Autodesk Inventor part; units mm, degrees
(part 2 of 2)
sketch "スケッチ3" plane through (0, 0, 0) normal (0, 0, 1) x (1, 0, 0)
  circle A0 centre (-65.3767, 79.8352) radius 5.25 projected
  arc A1 (-43.2653, 88.6866) -> (-43.9344, 87.9435) centre (-42.9563, 87.7355) ccw projected
  line L0 (-43.9344, 87.9435) -> (-47.1214, 72.9516) projected
  arc A2 (-47.1214, 72.9516) -> (-45.8786, 71.7794) centre (-46.1433, 72.7437) ccw projected
  arc A3 (-42.2436, 64.1319) -> (-45.8786, 71.7794) centre (-44.7404, 67.6327) ccw projected
  arc A4 (-42.2436, 64.1319) -> (-42.659, 63.2293) centre (-41.663, 63.3177) ccw projected
  arc A5 (-53.0468, 54.5405) -> (-42.659, 63.2293) centre (-50.8767, 62.5) ccw projected
  arc A6 (-53.0468, 54.5405) -> (-54.0085, 54.2911) centre (-53.3098, 53.5757) ccw projected
  arc A7 (-59.6272, 53.9531) -> (-54.0085, 54.2911) centre (-57.0131, 57.3673) ccw projected
  arc A8 (-59.6272, 53.9531) -> (-60.795, 53.9877) centre (-60.2351, 53.1591) ccw projected
  line L1 (-60.795, 53.9877) -> (-61.9497, 53.2074) projected
  arc A9 (-61.9497, 53.2074) -> (-62.3865, 52.4596) centre (-61.3898, 52.3788) ccw projected
  arc A10 (-68.3669, 52.4596) -> (-62.3865, 52.4596) centre (-65.3767, 52.702) ccw projected
  arc A11 (-68.3669, 52.4596) -> (-68.8038, 53.2074) centre (-69.3637, 52.3788) ccw projected
  line L2 (-68.8038, 53.2074) -> (-69.9585, 53.9877) projected
  arc A12 (-69.9585, 53.9877) -> (-71.1263, 53.9531) centre (-70.5184, 53.1591) ccw projected
  arc A13 (-76.7449, 54.2911) -> (-71.1263, 53.9531) centre (-73.7404, 57.3673) ccw projected
  arc A14 (-76.7449, 54.2911) -> (-77.7067, 54.5405) centre (-77.4437, 53.5757) ccw projected
  arc A15 (-88.0944, 63.2293) -> (-77.7067, 54.5405) centre (-79.8767, 62.5) ccw projected
  arc A16 (-88.0944, 63.2293) -> (-88.5099, 64.1319) centre (-89.0905, 63.3177) ccw projected
  arc A17 (-89.8355, 69.6024) -> (-88.5099, 64.1319) centre (-86.0131, 67.6327) ccw projected
  arc A18 (-89.8355, 69.6024) -> (-90.0078, 70.7579) centre (-90.7244, 70.0604) ccw projected
  line L3 (-90.0078, 70.7579) -> (-90.9798, 71.7565) projected
  arc A19 (-90.9798, 71.7565) -> (-91.7931, 72.0544) centre (-91.6964, 71.059) ccw projected
  arc A20 (-92.8499, 77.9406) -> (-91.7931, 72.0544) centre (-92.0829, 75.0403) ccw projected
  arc A21 (-92.8499, 77.9406) -> (-92.1911, 78.5027) centre (-93.1056, 78.9074) ccw projected
  line L4 (-92.1911, 78.5027) -> (-91.6272, 79.7771) projected
  arc A22 (-91.6272, 79.7771) -> (-91.8676, 80.9205) centre (-92.5416, 80.1818) ccw projected
  arc A23 (-92.5278, 86.5104) -> (-91.8676, 80.9205) centre (-88.9691, 84.0968) ccw projected
  arc A24 (-92.5278, 86.5104) -> (-92.4523, 87.5011) centre (-93.3554, 87.0717) ccw projected
  arc A25 (-85.7359, 99.2608) -> (-92.4523, 87.5011) centre (-85.0015, 91.0436) ccw projected
  arc A26 (-85.7359, 99.2608) -> (-84.921, 99.8292) centre (-85.8249, 100.2569) ccw projected
  arc A27 (-79.7708, 102.1007) -> (-84.921, 99.8292) centre (-81.034, 97.9904) ccw projected
  arc A28 (-79.7708, 102.1007) -> (-78.6639, 102.4745) centre (-79.4771, 103.0566) ccw projected
  line L5 (-78.6639, 102.4745) -> (-77.8528, 103.6077) projected
  arc A29 (-77.8528, 103.6077) -> (-77.7034, 104.4608) centre (-78.6659, 104.1898) ccw projected
  arc A30 (-72.0965, 106.5412) -> (-77.7034, 104.4608) centre (-74.8156, 105.2737) ccw projected
  arc A31 (-72.0965, 106.5412) -> (-71.4268, 105.9921) centre (-71.1901, 106.9637) ccw projected
  line L6 (-71.4268, 105.9921) -> (-70.0728, 105.6623) projected
  arc A32 (-70.0728, 105.6623) -> (-68.99, 106.1009) centre (-69.8361, 106.6338) ccw projected
  arc A33 (-63.6047, 107.7386) -> (-68.99, 106.1009) centre (-65.3514, 103.8094) ccw projected
  arc A34 (-63.6047, 107.7386) -> (-62.6162, 107.8393) centre (-63.1984, 108.6523) ccw projected
  arc A35 (-49.8547, 103.3068) -> (-62.6162, 107.8393) centre (-57.8128, 101.1319) ccw projected
  arc A36 (-49.8547, 103.3068) -> (-49.1512, 102.6051) centre (-48.89, 103.5704) ccw projected
  arc A37 (-46.0508, 97.6465) -> (-49.1512, 102.6051) centre (-50.2742, 98.4544) ccw projected
  arc A38 (-46.0508, 97.6465) -> (-44.9551, 96.465) centre (-45.0686, 97.4586) ccw projected
  arc A39 (-43.2653, 88.6866) -> (-44.9551, 96.465) centre (-44.5012, 92.4909) ccw projected
  arc A40 (-60.3905, 85.4377) -> (-59.2073, 85.3296) centre (-59.7257, 86.1847) ccw projected
  line L7 (-59.2073, 85.3296) -> (-48.9817, 91.5288) projected
  arc A41 (-48.9817, 91.5288) -> (-48.5003, 92.4053) centre (-49.5001, 92.3839) ccw projected
  arc A42 (-48.4958, 92.6994) -> (-48.5003, 92.4053) centre (-44.5012, 92.4909) ccw projected
  arc A43 (-48.4958, 92.6994) -> (-48.95, 93.5904) centre (-49.4944, 92.7516) ccw projected
  line L8 (-48.95, 93.5904) -> (-49.574, 93.9954) projected
  arc A44 (-49.574, 93.9954) -> (-50.1478, 94.1562) centre (-50.1185, 93.1567) ccw projected
  arc A45 (-52.021, 94.5252) -> (-50.1478, 94.1562) centre (-50.2742, 98.4544) ccw projected
  arc A46 (-52.021, 94.5252) -> (-53.0094, 94.4244) centre (-52.4272, 93.6114) ccw projected
  arc A47 (-65.771, 98.9569) -> (-53.0094, 94.4244) centre (-57.8128, 101.1319) ccw projected
  arc A48 (-65.771, 98.9569) -> (-66.4744, 99.6586) centre (-66.7356, 98.6933) ccw projected
  arc A49 (-69.2468, 101.9882) -> (-66.4744, 99.6586) centre (-65.3514, 103.8094) ccw projected
  arc A50 (-69.2468, 101.9882) -> (-69.916, 102.5363) centre (-70.1527, 101.5647) ccw projected
  line L9 (-69.916, 102.5363) -> (-70.5978, 102.7024) projected
  arc A51 (-70.5978, 102.7024) -> (-71.772, 101.383) centre (-70.8345, 101.7308) ccw projected
  line L10 (-71.772, 101.383) -> (-66.7965, 87.9737) projected
  arc A52 (-66.7965, 87.9737) -> (-65.8023, 87.3231) centre (-65.859, 88.3215) ccw projected
  arc A53 (-60.3905, 85.4377) -> (-65.8023, 87.3231) centre (-65.3767, 79.8352) ccw projected
  line L11 (-63.8767, 71.7112) -> (-63.8767, 57.4086) projected
  arc A54 (-63.8767, 57.4086) -> (-62.3169, 56.58) centre (-62.8767, 57.4086) ccw projected
  line L12 (-62.3169, 56.58) -> (-61.7354, 56.9729) projected
  arc A55 (-61.7354, 56.9729) -> (-61.2986, 57.7196) centre (-62.2953, 57.8015) ccw projected
  arc A56 (-59.5099, 60.8681) -> (-61.2986, 57.7196) centre (-57.0131, 57.3673) ccw projected
  arc A57 (-59.5099, 60.8681) -> (-59.0944, 61.7707) centre (-60.0905, 61.6823) ccw projected
  arc A58 (-51.4061, 70.733) -> (-59.0944, 61.7707) centre (-50.8767, 62.5) ccw projected
  arc A59 (-51.4061, 70.733) -> (-50.4921, 71.523) centre (-51.4703, 71.7309) ccw projected
  line L13 (-50.4921, 71.523) -> (-47.1705, 87.1482) projected
  arc A60 (-47.1705, 87.1482) -> (-48.6671, 88.2112) centre (-48.1487, 87.3561) ccw projected
  line L14 (-48.6671, 88.2112) -> (-58.3104, 82.365) projected
  arc A61 (-58.3494, 82.4556) -> (-58.3104, 82.365) centre (-57.4124, 82.805) ccw projected
  arc A62 (-63.1709, 72.667) -> (-58.3494, 82.4556) centre (-65.3767, 79.8352) ccw projected
  arc A63 (-63.1709, 72.667) -> (-63.8767, 71.7112) centre (-62.8767, 71.7112) ccw projected
  line L15 (-66.8767, 57.4086) -> (-66.8767, 71.7112) projected
  arc A64 (-66.8767, 71.7112) -> (-67.5826, 72.667) centre (-67.8767, 71.7112) ccw projected
  arc A65 (-72.0424, 76.3973) -> (-67.5826, 72.667) centre (-65.3767, 79.8352) ccw projected
  arc A66 (-72.0424, 76.3973) -> (-73.1078, 76.9232) centre (-72.9311, 75.9389) ccw projected
  line L16 (-73.1078, 76.9232) -> (-87.1853, 74.3957) projected
  arc A67 (-87.1853, 74.3957) -> (-87.7252, 72.7139) centre (-87.0086, 73.4114) ccw projected
  line L17 (-87.7252, 72.7139) -> (-87.2357, 72.211) projected
  arc A68 (-87.2357, 72.211) -> (-86.4237, 71.9131) centre (-86.5192, 72.9085) ccw projected
  arc A69 (-83.0085, 70.7089) -> (-86.4237, 71.9131) centre (-86.0131, 67.6327) ccw projected
  arc A70 (-83.0085, 70.7089) -> (-82.0468, 70.4595) centre (-82.3098, 71.4243) ccw projected
  arc A71 (-71.659, 61.7707) -> (-82.0468, 70.4595) centre (-79.8767, 62.5) ccw projected
  arc A72 (-71.659, 61.7707) -> (-71.2436, 60.8681) centre (-70.663, 61.6823) ccw projected
  arc A73 (-69.4548, 57.7196) -> (-71.2436, 60.8681) centre (-73.7404, 57.3673) ccw projected
  arc A74 (-69.4548, 57.7196) -> (-69.0181, 56.9729) centre (-68.4582, 57.8015) ccw projected
  line L18 (-69.0181, 56.9729) -> (-68.4366, 56.58) projected
  arc A75 (-68.4366, 56.58) -> (-66.8767, 57.4086) centre (-67.8767, 57.4086) ccw projected
  circle A76 centre (-74.8156, 105.2737) radius 1.5 projected
  circle A77 centre (-92.0829, 75.0403) radius 1.5 projected
  circle A78 centre (-85.0015, 91.0436) radius 5.25 projected
  circle A79 centre (-88.9691, 84.0968) radius 1.3 projected
  circle A80 centre (-81.034, 97.9904) radius 1.3 projected
  circle A81 centre (-65.3514, 103.8094) radius 1.3 projected
  circle A82 centre (-50.2742, 98.4544) radius 1.3 projected
  circle A83 centre (-57.8128, 101.1319) radius 5.25 projected
  circle A84 centre (-86.0131, 67.6327) radius 1.3 projected
  circle A85 centre (-79.8767, 62.5) radius 5.25 projected
  line L19 (-76.3353, 100.5735) -> (-76.7438, 100.0029) projected
  arc A86 (-76.7438, 100.0029) -> (-76.8935, 99.1509) centre (-75.9306, 99.4208) ccw projected
  arc A87 (-77.4753, 95.5768) -> (-76.8935, 99.1509) centre (-81.034, 97.9904) ccw projected
  arc A88 (-77.4753, 95.5768) -> (-77.5508, 94.5861) centre (-76.6477, 95.0154) ccw projected
  arc A89 (-84.2672, 82.8263) -> (-77.5508, 94.5861) centre (-85.0015, 91.0436) ccw projected
  arc A90 (-84.2672, 82.8263) -> (-85.0821, 82.2579) centre (-84.1781, 81.8303) ccw projected
  arc A91 (-87.865, 79.9409) -> (-85.0821, 82.2579) centre (-88.9691, 84.0968) ccw projected
  arc A92 (-87.865, 79.9409) -> (-88.5227, 79.3791) centre (-87.6082, 78.9744) ccw projected
  line L20 (-88.5227, 79.3791) -> (-88.8067, 78.7374) projected
  arc A93 (-88.8067, 78.7374) -> (-87.7155, 77.3484) centre (-87.8922, 78.3327) ccw projected
  line L21 (-87.7155, 77.3484) -> (-73.638, 79.876) projected
  arc A94 (-73.638, 79.876) -> (-72.822, 80.7396) centre (-73.8147, 80.8602) ccw projected
  arc A95 (-69.9385, 85.7884) -> (-72.822, 80.7396) centre (-65.3767, 79.8352) ccw projected
  arc A96 (-69.9385, 85.7884) -> (-69.6092, 86.93) centre (-70.5467, 86.5822) ccw projected
  line L22 (-69.6092, 86.93) -> (-74.5846, 100.3393) projected
  arc A97 (-74.5846, 100.3393) -> (-76.3353, 100.5735) centre (-75.5222, 99.9915) ccw projected
  circle A98 centre (-44.5012, 92.4909) radius 1.25 projected
  circle A99 centre (-65.3767, 52.702) radius 1.5 projected
  circle A100 centre (-57.0131, 57.3673) radius 1.3 projected
  circle A101 centre (-50.8767, 62.5) radius 5.25 projected
  circle A102 centre (-44.7404, 67.6327) radius 1.3 projected
  circle A103 centre (-73.7404, 57.3673) radius 1.3 projected
  circle A104 centre (-92.0829, 75.0403) radius 1.5 projected
  circle A105 centre (-92.0829, 75.0403) radius 3
  circle A106 centre (-88.9691, 84.0968) radius 1.3 projected
  arc A107 (-87.865, 79.9409) -> (-85.0821, 82.2579) centre (-88.9691, 84.0968) ccw projected
  circle A108 centre (-88.9691, 84.0968) radius 4.3
  circle A109 centre (-86.0131, 67.6327) radius 1.3 projected
  arc A110 (-83.0085, 70.7089) -> (-86.4237, 71.9131) centre (-86.0131, 67.6327) ccw projected
  circle A111 centre (-86.0131, 67.6327) radius 4.3
  circle A112 centre (-81.034, 97.9904) radius 1.3 projected
  arc A113 (-76.7438, 100.0029) -> (-76.8935, 99.1509) centre (-75.9306, 99.4208) ccw projected
  circle A114 centre (-81.034, 97.9904) radius 4.3
  circle A115 centre (-73.7404, 57.3673) radius 4.3
  arc A116 (-68.3669, 52.4596) -> (-62.3865, 52.4596) centre (-65.3767, 52.702) ccw projected
  circle A117 centre (-65.3767, 52.702) radius 3
  arc A118 (-59.6272, 53.9531) -> (-54.0085, 54.2911) centre (-57.0131, 57.3673) ccw projected
  circle A119 centre (-57.0131, 57.3673) radius 4.3
  arc A120 (-43.2653, 88.6866) -> (-44.9551, 96.465) centre (-44.5012, 92.4909) ccw projected
  circle A121 centre (-44.5012, 92.4909) radius 4
  arc A122 (-72.0965, 106.5412) -> (-77.7034, 104.4608) centre (-74.8156, 105.2737) ccw projected
  circle A123 centre (-74.8156, 105.2737) radius 3
  arc A124 (-70.0728, 105.6623) -> (-68.99, 106.1009) centre (-69.8361, 106.6338) ccw projected
  circle A125 centre (-65.3514, 103.8094) radius 4.3
  line L23 (-85.0015, 91.0436) -> (-74.8156, 105.2737) construction
  line L24 (-83.7818, 90.1705) -> (-73.5959, 104.4006)
  line L25 (-76.0353, 106.1468) -> (-86.2213, 91.9167)
  arc A126 (-86.2213, 91.9167) -> (-83.7818, 90.1705) centre (-85.0015, 91.0436) ccw
  arc A127 (-73.5959, 104.4006) -> (-76.0353, 106.1468) centre (-74.8156, 105.2737) ccw
  line L26 (-74.8156, 105.2737) -> (-57.8128, 101.1319) construction
  line L27 (-75.1706, 103.8163) -> (-58.1678, 99.6745)
  line L28 (-57.4578, 102.5892) -> (-74.4606, 106.7311)
  arc A128 (-74.4606, 106.7311) -> (-75.1706, 103.8163) centre (-74.8156, 105.2737) ccw
  arc A129 (-58.1678, 99.6745) -> (-57.4578, 102.5892) centre (-57.8128, 101.1319) ccw
  line L29 (-57.8128, 101.1319) -> (-44.5012, 92.4909) construction
  line L30 (-58.6295, 99.8737) -> (-45.318, 91.2327)
  line L31 (-43.6845, 93.749) -> (-56.9961, 102.39)
  arc A130 (-56.9961, 102.39) -> (-58.6295, 99.8737) centre (-57.8128, 101.1319) ccw
  arc A131 (-45.318, 91.2327) -> (-43.6845, 93.749) centre (-44.5012, 92.4909) ccw
  line L32 (-44.5012, 92.4909) -> (-50.8767, 62.5) construction
  line L33 (-45.9685, 92.8028) -> (-52.344, 62.8119)
  line L34 (-49.4095, 62.1881) -> (-43.034, 92.179)
  arc A132 (-43.034, 92.179) -> (-45.9685, 92.8028) centre (-44.5012, 92.4909) ccw
  arc A133 (-52.344, 62.8119) -> (-49.4095, 62.1881) centre (-50.8767, 62.5) ccw
  line L35 (-79.8767, 62.5) -> (-65.3767, 52.702) construction
  line L36 (-80.7166, 61.2571) -> (-66.2166, 51.4592)
  line L37 (-64.5369, 53.9449) -> (-79.0369, 63.7429)
  arc A134 (-79.0369, 63.7429) -> (-80.7166, 61.2571) centre (-79.8767, 62.5) ccw
  arc A135 (-66.2166, 51.4592) -> (-64.5369, 53.9449) centre (-65.3767, 52.702) ccw
  line L38 (-65.3767, 52.702) -> (-50.8767, 62.5) construction
  line L39 (-64.5369, 51.4592) -> (-50.0369, 61.2571)
  line L40 (-51.7166, 63.7429) -> (-66.2166, 53.9449)
  arc A136 (-66.2166, 53.9449) -> (-64.5369, 51.4592) centre (-65.3767, 52.702) ccw
  arc A137 (-50.0369, 61.2571) -> (-51.7166, 63.7429) centre (-50.8767, 62.5) ccw
  line L41 (-85.0015, 91.0436) -> (-92.0829, 75.0403) construction
  line L42 (-86.3732, 91.6506) -> (-93.4546, 75.6473)
  line L43 (-90.7112, 74.4334) -> (-83.6298, 90.4366)
  arc A138 (-83.6298, 90.4366) -> (-86.3732, 91.6506) centre (-85.0015, 91.0436) ccw
  arc A139 (-93.4546, 75.6473) -> (-90.7112, 74.4334) centre (-92.0829, 75.0403) ccw
  line L44 (-86.0131, 67.6327) -> (-92.0829, 75.0403) construction
  line L45 (-84.8529, 68.5834) -> (-90.9226, 75.991)
  line L46 (-93.2431, 74.0896) -> (-87.1733, 66.682)
  arc A140 (-87.1733, 66.682) -> (-84.8529, 68.5834) centre (-86.0131, 67.6327) ccw
  arc A141 (-90.9226, 75.991) -> (-93.2431, 74.0896) centre (-92.0829, 75.0403) ccw
  point P0 (0, 0)
  point P1 (-79.9086, 98.1587)
  point P2 (-66.3142, 103.2028)
  point P3 (-51.157, 96.8114)
  point P4 (-47.689, 77.4954)
  point P5 (-72.6267, 57.601)
  point P6 (-58.1267, 57.601)
  point P7 (-88.5422, 83.042)
  point P8 (-89.048, 71.3365)
  point P9 (-66.6896, 55.3995)
  point P10 (-64.0639, 55.3995)
  point P11 (-46.7395, 89.1757)
  point P12 (-72.6464, 103.2014)
  point P13 (-75.1081, 102.288)
  point P14 (-89.6599, 76.8092)
  point P15 (-89.276, 73.9814)
  point P16 (-87.407, 71.7005)
  dimension "d9" = 3
  dimension "d10" = 3
  dimension "d11" = 3
  dimension "d12" = 3
  dimension "d13" = 3
  dimension "d14" = 3
  dimension "d15" = 3
  dimension "d16" = 3
  constraints: 64 end point, 32 point on circle, 32 tangent, 16 centre point, 11 coincident, 8 midpoint, 8 parallel, 4 concentric, 30 other
  measures "d9" diameter of A127
  measures "d10" diameter of A129
  measures "d11" diameter of A131
  measures "d12" diameter of A133
  measures "d13" diameter of A135
  measures "d14" diameter of A137
  measures "d15" diameter of A139
  measures "d16" diameter of A141
extrude "押し出し3" cut sketch "スケッチ3" against normal blind 10 contours A0 | L33 A60 L14 A61 A62 A63 L11 A54 L40 A117 L37 A75 L15 A64 A65 A66 L16 A67 L17 A68 A111 L45 A105 L43 A93 L21 A94 A95 A96 L22 A97 L24 A123 L27 A51 L10 A52 A53 A40 L7 A41 A121
fillet "フィレット2" radius 1 7 edges at (-89.276, 73.9814, -2) (-89.6599, 76.8092, -2) (-72.6464, 103.2014, -2) (-75.1081, 102.288, -2) (-46.7395, 89.1757, -2) (-64.0639, 55.3995, -2) (-66.6896, 55.3995, -2)
